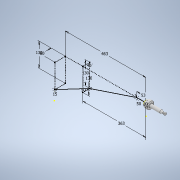
# Autodesk Inventor part: 78. Рычаг переключения
Saved by Autodesk Inventor 2021 (Build 250183000, 183)
## iProperties
Created: 2021-03-18
Part Number: 78. Рычаг переключения
Material: Типовые
Document SubType Name: Modeling
Designer: Данил
Density: 1 g/cm^3
Appearance: По умолчанию
Author: Данил
Autodesk Inventor part; units mm, degrees
ref_plane "YZ Plane" through (0, 0, 0) normal (1, 0, 0) x (0, 1, 0)
ref_plane "XZ Plane" through (0, 0, 0) normal (0, 1, 0) x (-1, 0, 0)
ref_plane "XY Plane" through (0, 0, 0) normal (0, 0, 1) x (1, 0, 0)
sketch "Эскиз1" plane through (0, 0, 0) normal (0, 0, 1) x (1, 0, 0)
  line L0 (-288.5, 0) -> (288.5, 0) construction
  line L1 (0, 67.5) -> (0, -67.5) construction
  arc A0 (288.5, 72.399) -> (278.9977, 72.86) centre (283.5, 67.5) ccw
  line L2 (288.5, 67.5) -> (288.5, 72.399)
  line L3 (174.5, 67.5) -> (288.5, 67.5)
  arc A1 (273.5, 72) -> (278.9977, 72.86) centre (275.5372, 76.9797) ccw
  line L4 (273.5, 72) -> (262.5, 76.5)
  line L5 (262.5, 76.5) -> (202.5, 76.5)
  line L6 (200.5, 78.5) -> (200.5, 87.3006)
  arc A2 (200.5, 78.5) -> (202.5, 76.5) centre (202.5, 78.5) ccw
  arc A3 (200.5, 87.3006) -> (174.5, 81.067) centre (191.5, 67.5) ccw
  line L7 (174.5, 81.067) -> (174.5, 67.5)
  point P0 (0, 0)
  point P1 (0, 0)
  dimension "d0" = 577
  dimension "d1" = 135
  dimension "d2" = 14
  dimension "d3" = 5
  dimension "d4" = 9
  dimension "d5" = 26
  dimension "d6" = 18
  dimension "d9" = 2
  dimension "d12" = 10
  dimension "d14" = 43.5
  dimension "d15" = 26
  dimension "d16" = 114
  dimension "d17" = 17
  constraints: 17 end point, 8 point on circle, 4 centre point, 4 tangent, 4 vertical, 3 horizontal alignment, 2 horizontal, 2 midpoint, 2 vertical alignment, 1 coincident, 1 point on line
  measures "d0" distance of L0.start L0.end
  measures "d1" distance of L1.start L1.end
  measures "d2" diameter of A0
  measures "d3" horizontal distance of L0.end A0.centre
  measures "d4" diameter of L4.start L3
  measures "d5" distance from line of L2 L4.end
  measures "d6" diameter of L5 L3
  measures "d9" radius of A2
  measures "d12" horizontal distance of L4.start A0.centre
  measures "d14" diameter of A3
  measures "d15" distance between parallel lines of L7 L6
  measures "d16" distance between parallel lines of L7 L2
  measures "d17" distance from line of L7 A3.centre
revolve "Вращение1" add sketch "Эскиз1" angle 360 about axis through (174.5, 67.5, 0) along (1, 0, 0)
sketch "Эскиз2" plane through (0, 0, 0) normal (0, 1, 0) x (-1, 0, 0)
  line L0 (-275.5372, 14.5) -> (-288.5, 14.5)
  line L1 (-288.5, 14.5) -> (-288.5, 4.5)
  line L2 (-288.5, 4.5) -> (-275.5372, 4.5)
  line L3 (-275.5372, 4.5) -> (-275.5372, 14.5)
  line L4 (-275.5372, -14.5) -> (-288.5, -14.5)
  line L5 (-288.5, -14.5) -> (-288.5, -4.5)
  line L6 (-288.5, -4.5) -> (-275.5372, -4.5)
  line L7 (-275.5372, -4.5) -> (-275.5372, -14.5)
  line L8 (-282.0186, -4.5) -> (-282.0186, 4.5) construction
  arc A0 (-278.9977, 5.36) -> (-273.5, 4.5) centre (-275.5372, 9.4797) ccw projected
  line L9 (-288.5, 4.899) -> (-288.5, -4.899) projected
  point P0 (0, 0)
  point P1 (-282.0186, 0)
  point P2 (-288.5, 0)
  dimension "d19" = 9
  dimension "d20" = 10
  constraints: 18 end point, 4 midpoint, 4 parallel, 2 horizontal, 2 perpendicular, 2 vertical alignment, 1 collinear, 1 horizontal alignment, 1 point on line, 1 vertical
  measures "d19" distance of L8.start L8.end
  measures "d20" distance of L0.end L1.end
extrude "Выдавливание1" cut sketch "Эскиз2" along normal through all
sketch "Эскиз3" plane through (200.5, 67.5, 0) normal (1, 0, 0) x (0, 0, -1)
  circle A0 centre (0, 0) radius 21.75 projected
  line L0 (-21.75, 3.25) -> (-15, 3.25)
  line L1 (-15, 3.25) -> (-15, -3.25)
  line L2 (-15, -3.25) -> (-21.75, -3.25)
  line L3 (-21.75, -3.25) -> (-21.75, 3.25)
  line L4 (15, 3.25) -> (21.75, 3.25)
  line L5 (21.75, 3.25) -> (21.75, -3.25)
  line L6 (21.75, -3.25) -> (15, -3.25)
  line L7 (15, -3.25) -> (15, 3.25)
  line L8 (-15, 0) -> (15, 0) construction
  point P0 (0, -67.5)
  point P1 (21.5058, -3.25)
  point P2 (21.5058, 3.25)
  point P3 (-21.5058, 3.25)
  point P4 (-21.5058, -3.25)
  dimension "d23" = 30
  dimension "d24" = 6.5
  constraints: 18 end point, 4 parallel, 3 midpoint, 2 horizontal, 2 perpendicular, 2 point on line, 2 tangent, 1 coincident
  measures "d23" distance of L8.start L8.end
  measures "d24" distance of L4.end L5.end
extrude "Выдавливание2" cut sketch "Эскиз3" against normal through all both and the other way through all contours A0 L6 L7 L4 | L0 L1 L2 A0
sketch3d "3D эскиз1"
sketch "Эскиз8" plane through (174.5, 67.5, 0) normal (-1, 0, 0) x (0, 0, 1)
  circle A0 centre (0, 0) radius 10
  point P0 (0, -67.5)
  dimension "d57" = 20
  constraints: 1 centre point, 1 coincident
  measures "d57" diameter of A0
ref_plane "РабПлоскость4" through (-288.5, -67.5, 60) normal (-0.7066653, -0.0353333, 0.7066653) x (0.0499376, -0.9987523, 0)
sketch "Эскиз9" plane through (-288.5, -67.5, 60) normal (-0.7066653, -0.0353333, 0.7066653) x (0.0499376, -0.9987523, 0)
  circle A0 centre (0, 0) radius 7.5
  point P0 (-53.0088, 163.5477)
  dimension "d58" = 15
  constraints: 1 centre point, 1 coincident
  measures "d58" diameter of A0
